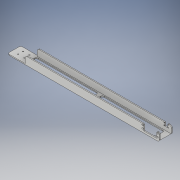
# Autodesk Inventor part: ArmProto1.2
Saved by Autodesk Inventor 2017 (Build 210142000, 142)
## iProperties
Created: 2017-09-30
Part Number: ArmProto1.2
Material: Generic
Document SubType Name: Modeling
Designer: User
Density: 1 g/cm^3
Appearance: Default
Author: User
Autodesk Inventor part; units mm, degrees
ref_plane "YZ Plane" through (0, 0, 0) normal (1, 0, 0) x (0, 1, 0)
ref_plane "XZ Plane" through (0, 0, 0) normal (0, 1, 0) x (-1, 0, 0)
ref_plane "XY Plane" through (0, 0, 0) normal (0, 0, 1) x (1, 0, 0)
sketch "Sketch1" plane through (0, 0, 0) normal (1, 0, 0) x (0, 1, 0)
  line L0 (0, 0) -> (25.4, 0)
  line L1 (25.4, 0) -> (25.4, -42.799)
  line L2 (25.4, -42.799) -> (0, -42.799)
  line L3 (0, -42.799) -> (0, 0)
  line L4 (25.4, -3.175) -> (3.175, -3.175)
  line L5 (3.175, -3.175) -> (3.175, -39.624)
  line L6 (3.175, -39.624) -> (25.4, -39.624)
  line L7 (25.4, -39.624) -> (25.4, -3.175)
  dimension "d0" = 25.4
  dimension "d1" = 42.799
  dimension "d2" = 22.225
  dimension "d3" = 36.449
  dimension "d4" = 3.175
  constraints: 16 end point, 4 parallel, 2 horizontal, 2 perpendicular, 1 point on line
  measures "d0" distance of L1.end L2.end
  measures "d1" distance of L0.end L1.end
  measures "d2" distance of L5.end L6.end
  measures "d3" distance of L4.end L5.end
  measures "d4" distance between parallel lines of L0 L4
extrude "Extrusion1" add sketch "Sketch1" along normal blind 495.3 contours L0 L1 L4 L5 L6 L2 L3
sketch "Sketch2" plane through (0, 0, 0) normal (0, 0, 1) x (1, 0, 0)
  line L0 (0, 25.4) -> (0, 0) projected
  line L1 (0, 0) -> (495.3, 0) projected
  line L2 (495.3, 25.4) -> (495.3, 0) projected
  line L3 (0, 25.4) -> (495.3, 25.4) projected
  line L4 (486.41, 25.4) -> (444.5, 25.4)
  line L5 (444.5, 25.4) -> (444.5, 6.35)
  line L6 (444.5, 6.35) -> (486.41, 6.35)
  line L7 (486.41, 6.35) -> (486.41, 25.4)
  circle A0 centre (490.2962, 21.2344) radius 2.413
  circle A1 centre (490.2962, 11.2344) radius 2.413
  circle A2 centre (440.7962, 21.2344) radius 2.413
  circle A3 centre (440.7962, 11.2344) radius 2.413
  dimension "d7" = 8.89
  dimension "d8" = 25.4
  dimension "d9" = 19.05
  dimension "d10" = 50.8
  dimension "d11" = 4.826
  dimension "d12" = 4.826
  dimension "d13" = 4.1656
  dimension "d14" = 10
  dimension "d15" = 4.826
  dimension "d16" = 4.826
  dimension "d26" = 5.0038
  dimension "d27" = 5.0038
  dimension "d28" = 49.5
  dimension "d29" = 49.5
  dimension "d30" = 10
  constraints: 8 end point, 4 centre point, 2 parallel, 1 horizontal, 1 perpendicular, 1 point on line
  measures "d7" distance between parallel lines of L2 L7
  measures "d8" distance of L2.start L1.end
  measures "d9" distance of L6.end L4.start
  measures "d10" distance between parallel lines of L2 L5
  measures "d11" diameter of A0
  measures "d12" diameter of A1
  measures "d13" distance from line of A0.centre L3
  measures "d14" distance of A1.centre A0.centre
  measures "d15" diameter of A2
  measures "d16" diameter of A3
  measures "d26" distance from line of L2 A0.centre
  measures "d27" distance from line of L2 A1.centre
  measures "d28" distance of A0.centre A2.centre
  measures "d29" distance of A1.centre A3.centre
  measures "d30" distance of A3.centre A2.centre
extrude "Extrusion2" cut sketch "Sketch2" against normal blind 12.7 contours L3 L7 L6 L5 | A0 | A1 | A2 | A3
fillet "Fillet1" radius 3.175 3 edges at (495.3, 25.4, -1.5875) (486.41, 25.4, -1.5875) (444.5, 25.4, -1.5875)
fillet "Fillet2" radius 6.35 2 edges at (495.3, 25.4, -41.2115) (495.3, 0, -21.3995)
sketch "Sketch6" plane through (0, 0, 0) normal (0, 0, 1) x (1, 0, 0)
  circle A0 centre (440.7962, 11.2344) radius 2.413 projected
  circle A1 centre (490.2962, 11.2344) radius 2.413 projected
  circle A2 centre (490.2962, 21.2344) radius 2.413 projected
  circle A3 centre (440.7962, 21.2344) radius 2.413 projected
  arc A4 (488.95, 0) -> (495.3, 6.35) centre (488.95, 6.35) ccw projected
  line L0 (495.3, 22.225) -> (495.3, 6.35) projected
  arc A5 (495.3, 22.225) -> (492.125, 25.4) centre (492.125, 22.225) ccw projected
  line L1 (489.585, 25.4) -> (492.125, 25.4) projected
  arc A6 (489.585, 25.4) -> (486.41, 22.225) centre (489.585, 22.225) ccw projected
  line L2 (486.41, 22.225) -> (486.41, 6.35) projected
  line L3 (486.41, 6.35) -> (444.5, 6.35) projected
  line L4 (444.5, 6.35) -> (444.5, 22.225) projected
  arc A7 (444.5, 22.225) -> (441.325, 25.4) centre (441.325, 22.225) ccw projected
  line L5 (0, 25.4) -> (441.325, 25.4) projected
  line L6 (0, 25.4) -> (0, 0) projected
  line L7 (0, 0) -> (488.95, 0) projected
  line L8 (0, 25.4) -> (57.15, 25.4)
  line L9 (57.15, 25.4) -> (57.15, 3.175)
  line L10 (57.15, 3.175) -> (0, 3.175)
  line L11 (0, 3.175) -> (0, 25.4)
  dimension "d46" = 57.15
  dimension "d47" = 22.225
  constraints: 8 end point, 2 parallel, 1 horizontal, 1 perpendicular
  measures "d46" distance of L9.end L10.end
  measures "d47" distance of L8.end L9.end
extrude "Extrusion5" cut sketch "Sketch6" against normal blind 127 contours L6 L5 L9 L10
fillet "Fillet3" radius 6.35 4 edges at (57.15, 25.4, -1.5875) (57.15, 25.4, -41.2115) (0, 1.5875, 0) (0, 1.5875, -42.799)
sketch "Sketch7" plane through (488.95, 0, -42.799) normal (0, -1, 0) x (1, 0, 0)
  arc A0 (-488.95, 6.35) -> (-482.6, 0) centre (-482.6, 6.35) ccw projected
  line L0 (-482.6, 0) -> (0, 0) projected
  line L1 (0, 42.799) -> (0, 0) projected
  line L2 (-482.6, 42.799) -> (0, 42.799) projected
  arc A1 (-482.6, 42.799) -> (-488.95, 36.449) centre (-482.6, 36.449) ccw projected
  line L3 (-488.95, 36.449) -> (-488.95, 6.35) projected
  line L4 (-431.8, 36.449) -> (-228.6, 36.449)
  line L5 (-228.6, 36.449) -> (-228.6, 6.35)
  line L6 (-228.6, 6.35) -> (-431.8, 6.35)
  line L7 (-431.8, 6.35) -> (-431.8, 36.449)
  line L8 (-215.9, 36.449) -> (-12.7, 36.449)
  line L9 (-12.7, 36.449) -> (-12.7, 6.35)
  line L10 (-12.7, 6.35) -> (-215.9, 6.35)
  line L11 (-215.9, 6.35) -> (-215.9, 36.449)
  point P0 (-488.95, 42.799)
  dimension "d52" = 42.799
  dimension "d53" = 6.35
  dimension "d54" = 6.35
  dimension "d55" = 57.15
  dimension "d56" = 431.8
  dimension "d57" = 203.2
  dimension "d58" = 203.2
  dimension "d59" = 6.35
  dimension "d60" = 6.35
  dimension "d61" = 12.7
  constraints: 16 end point, 4 parallel, 2 horizontal, 2 perpendicular
  measures "d52" distance of L1.start L0.end
  measures "d53" distance between parallel lines of L2 L4
  measures "d54" distance between parallel lines of L0 L6
  measures "d55" distance between parallel lines of L3 L7
  measures "d56" distance between parallel lines of L1 L7
  measures "d57" distance of L4.start L4.end
  measures "d58" distance of L8.start L8.end
  measures "d59" distance between parallel lines of L2 L8
  measures "d60" distance between parallel lines of L0 L10
  measures "d61" distance between parallel lines of L5 L11
extrude "Extrusion6" cut sketch "Sketch7" against normal blind 127 contours L4 L5 L6 L7 | L8 L9 L10 L11
fillet "Fillet4" radius 6.35 8 edges at (260.35, 1.5875, -6.35) (57.15, 1.5875, -6.35) (57.15, 1.5875, -36.449) (273.05, 1.5875, -36.449) (273.05, 1.5875, -6.35) (260.35, 1.5875, -36.449) (476.25, 1.5875, -36.449) (476.25, 1.5875, -6.35)
sketch "Sketch8" plane through (494.4493, 3.175, -3.175) normal (0, 1, 0) x (1, 0, 0)
  line L0 (-437.2993, 9.525) -> (-437.2993, 26.924) projected
  arc A0 (-430.9493, 33.274) -> (-437.2993, 26.924) centre (-430.9493, 26.924) ccw projected
  line L1 (-430.9493, 33.274) -> (-240.4493, 33.274) projected
  arc A1 (-234.0993, 26.924) -> (-240.4493, 33.274) centre (-240.4493, 26.924) ccw projected
  line L2 (-234.0993, 26.924) -> (-234.0993, 9.525) projected
  arc A2 (-240.4493, 3.175) -> (-234.0993, 9.525) centre (-240.4493, 9.525) ccw projected
  line L3 (-240.4493, 3.175) -> (-430.9493, 3.175) projected
  arc A3 (-437.2993, 9.525) -> (-430.9493, 3.175) centre (-430.9493, 9.525) ccw projected
  line L4 (-221.3993, 9.525) -> (-221.3993, 26.924) projected
  arc A4 (-215.0493, 33.274) -> (-221.3993, 26.924) centre (-215.0493, 26.924) ccw projected
  line L5 (-215.0493, 33.274) -> (-24.5493, 33.274) projected
  arc A5 (-18.1993, 26.924) -> (-24.5493, 33.274) centre (-24.5493, 26.924) ccw projected
  line L6 (-18.1993, 26.924) -> (-18.1993, 9.525) projected
  arc A6 (-24.5493, 3.175) -> (-18.1993, 9.525) centre (-24.5493, 9.525) ccw projected
  line L7 (-24.5493, 3.175) -> (-215.0493, 3.175) projected
  arc A7 (-221.3993, 9.525) -> (-215.0493, 3.175) centre (-215.0493, 9.525) ccw projected
  arc A8 (-488.0993, 39.624) -> (-494.4493, 33.274) centre (-488.0993, 33.274) ccw projected
  line L8 (-494.4493, 3.175) -> (-494.4493, 33.274) projected
  arc A9 (-494.4493, 3.175) -> (-488.0993, -3.175) centre (-488.0993, 3.175) ccw projected
  line L9 (-437.2993, -3.175) -> (-488.0993, -3.175) projected
  line L10 (-437.2993, -3.175) -> (-437.2993, 0) projected
  line L11 (-437.2993, 0) -> (0, 0) projected
  line L12 (0, 36.449) -> (0, 0) projected
  line L13 (-437.2993, 36.449) -> (0, 36.449) projected
  line L14 (-437.2993, 36.449) -> (-437.2993, 39.624) projected
  line L15 (-488.0993, 39.624) -> (-437.2993, 39.624) projected
  line L16 (-474.6743, 27.504) -> (-454.2243, 27.504)
  line L17 (-454.2243, 27.504) -> (-454.2243, 11.504)
  line L18 (-454.2243, 11.504) -> (-474.6743, 11.504)
  line L19 (-474.6743, 11.504) -> (-474.6743, 27.504)
  point P0 (-494.4493, -3.175)
  dimension "d70" = 20.45
  dimension "d71" = 16
  dimension "d72" = 12.12
  dimension "d73" = 19.775
  constraints: 8 end point, 4 coincident, 2 parallel, 1 horizontal, 1 perpendicular
  measures "d70" distance of L17.end L18.end
  measures "d71" distance of L16.end L17.end
  measures "d72" distance between parallel lines of L15 L16
  measures "d73" distance between parallel lines of L8 L19
hole "Hole1" at (19.775, 3.175, -30.679) at (40.225, 3.175, -30.679) at (40.225, 3.175, -14.679) at (19.775, 3.175, -14.679) direction (0, -1, 0) diameter 3.7 depth 25.4 tip angle 118
sketch "Sketch9" plane through (495.3, 6.35, -42.799) normal (0, 0, -1) x (-1, 0, 0)
  line L0 (488.95, -3.175) -> (488.95, -6.35) projected
  line L1 (488.95, -3.175) -> (438.15, -3.175) projected
  line L2 (438.15, -3.175) -> (438.15, 12.7) projected
  arc A0 (438.15, 12.7) -> (431.8, 19.05) centre (431.8, 12.7) ccw projected
  line L3 (431.8, 19.05) -> (6.35, 19.05) projected
  arc A1 (6.35, 19.05) -> (0, 12.7) centre (6.35, 12.7) ccw projected
  line L4 (0, 0) -> (0, 12.7) projected
  arc A2 (0, 0) -> (6.35, -6.35) centre (6.35, 0) ccw projected
  line L5 (488.95, -6.35) -> (6.35, -6.35) projected
  circle A3 centre (9.5504, 9.4234) radius 1.2319
  circle A4 centre (23.4188, 9.4234) radius 1.2319
  circle A5 centre (23.4188, 17.4244) radius 1.2319
  circle A6 centre (9.5504, 17.4244) radius 1.2319
  line L6 (21.4846, 19.05) -> (11.4846, 19.05)
  line L7 (11.4846, 19.05) -> (11.4846, 8.3058)
  line L8 (11.4846, 8.3058) -> (21.4846, 8.3058)
  line L9 (21.4846, 8.3058) -> (21.4846, 19.05)
  point P0 (495.3, -6.35)
  dimension "d97" = 2.4638
  dimension "d98" = 2.4638
  dimension "d99" = 2.4638
  dimension "d100" = 2.4638
  dimension "d101" = 9.5504
  dimension "d102" = 9.5504
  dimension "d103" = 13.8684
  dimension "d104" = 13.8684
  dimension "d105" = 23.7744
  dimension "d106" = 15.7734
  dimension "d107" = 15.7734
  dimension "d108" = 23.7744
  dimension "d109" = 10
  dimension "d110" = 10.7442
  dimension "d111" = 1.9342
  constraints: 8 end point, 4 centre point, 2 parallel, 1 horizontal, 1 perpendicular, 1 point on line
  measures "d97" diameter of A3
  measures "d98" diameter of A4
  measures "d99" diameter of A5
  measures "d100" diameter of A6
  measures "d101" distance from line of L4 A3.centre
  measures "d102" distance from line of L4 A6.centre
  measures "d103" distance of A4.centre A3.centre
  measures "d104" distance of A5.centre A6.centre
  measures "d105" distance from line of L5 A6.centre
  measures "d106" distance from line of L5 A3.centre
  measures "d107" distance from line of L5 A4.centre
  measures "d108" distance from line of L5 A5.centre
  measures "d109" distance of L8.end L7.end
  measures "d110" distance of L8.end L6.start
  measures "d111" distance from line of L7 A6.centre
extrude "Extrusion7" cut sketch "Sketch9" against normal blind 6.35 contours L9 L8 L7 L3 | A3 | A4 | A5 | A6
equation "\"d12\" = d11"
equation "\"d15\" = d11"
equation "\"d16\" = d11"
equation "\"d27\" = d26"
equation "\"d29\" = d28"
equation "\"d30\" = d14"
equation "\"d58\" = d57"
equation "\"d98\" = d97"
equation "\"d99\" = d97"
equation "\"d100\" = d97"
equation "\"d102\" = d101"
equation "\"d104\" = d103"
equation "\"d107\" = d106"
equation "\"d108\" = d105"
equation "\"d111\" = -0.5 * d109 + 0.5 * d103"
body "Solid1"
